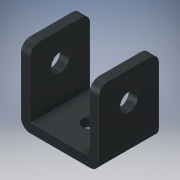
# Autodesk Inventor part: linear_actuator_connector
Saved by Autodesk Inventor 2019.4 (Build 234330000, 330)
## iProperties
Created: 2020-09-27
Part Number: linear_actuator_connector
Material: Iron, Cast
Document SubType Name: Modeling
Designer: deanv
Density: 7.15 g/cm^3
Appearance: Iron Gray
Author: deanv
Autodesk Inventor part; units mm, degrees
ref_plane "YZ Plane" through (0, 0, 0) normal (1, 0, 0) x (0, 1, 0)
ref_plane "XZ Plane" through (0, 0, 0) normal (0, 1, 0) x (-1, 0, 0)
ref_plane "XY Plane" through (0, 0, 0) normal (0, 0, 1) x (1, 0, 0)
sketch "Sketch1" plane through (0, 0, 0) normal (0, 0, 1) x (1, 0, 0)
  line L0 (-13, -12.5) -> (13, -12.5) construction
  line L1 (13, -12.5) -> (13, 12.5) construction
  line L2 (13, 12.5) -> (-13, 12.5) construction
  line L3 (-13, 12.5) -> (-13, -12.5) construction
  line L4 (-13, -12.5) -> (13, 12.5) construction
  line L5 (13, -12.5) -> (-13, 12.5) construction
  line L6 (-10, 12.5) -> (10, 12.5) construction
  line L7 (10, 12.5) -> (10, -9.5) construction
  line L8 (10, -9.5) -> (-10, -9.5) construction
  line L9 (-10, -9.5) -> (-10, 12.5) construction
  line L10 (-10, 12.5) -> (-13, 12.5)
  line L11 (-13, 12.5) -> (-13, -12.5)
  line L12 (-13, -12.5) -> (13, -12.5)
  line L13 (13, -12.5) -> (13, 12.5)
  line L14 (13, 12.5) -> (10, 12.5)
  line L15 (10, 12.5) -> (10, -9.5)
  line L16 (10, -9.5) -> (-10, -9.5)
  line L17 (-10, -9.5) -> (-10, 12.5)
  point P0 (0, 0)
  dimension "d0" = 26
  dimension "d1" = 25
  dimension "d2" = 3
  dimension "d3" = 3
  dimension "d4" = 3
  constraints: 36 end point, 5 collinear, 5 perpendicular, 4 parallel, 2 horizontal, 2 midpoint, 1 point on line
  measures "d0" distance of L2.end L1.end
  measures "d1" distance of L1.end L0.end
  measures "d2" distance between parallel lines of L3 L9
  measures "d3" distance between parallel lines of L1 L7
  measures "d4" distance between parallel lines of L0 L8
extrude "Extrusion1" add sketch "Sketch1" along normal blind 20
sketch "Sketch2" plane through (13, -12.5, 0) normal (1, 0, 0) x (0, 0, -1)
  line L0 (-20, 25) -> (-20, 0) construction
  line L1 (0, 0) -> (0, 25) construction
  line L2 (-20, 25) -> (0, 25) construction
  line L3 (0, 25) -> (0, 5) construction
  line L4 (0, 5) -> (-20, 5) construction
  line L5 (-20, 5) -> (-20, 25) construction
  line L6 (-20, 25) -> (0, 5) construction
  line L7 (-20, 5) -> (0, 25) construction
  line L8 (0, 25) -> (-20, 25) construction
  line L9 (-10, 25) -> (-10, 5) construction
  circle A0 centre (-10, 15.5) radius 3
  line L10 (0, 25) -> (0, 0) projected
  line L11 (-20, 0) -> (0, 0) construction
  line L12 (0, 0) -> (0, 3) construction
  line L13 (0, 3) -> (-20, 3) construction
  line L14 (-20, 3) -> (-20, 0) construction
  point P0 (0, 12.5)
  dimension "d7" = 20
  dimension "d17" = 6
  dimension "d20" = 3
  dimension "d21" = 12.5
  constraints: 22 end point, 4 parallel, 3 point on line, 2 horizontal, 2 midpoint, 2 perpendicular, 1 centre point
  measures "d7" distance of L2.end L3.end
  measures "d17" diameter of A0
  measures "d20" distance of L12.end L11.end
  measures "d21" distance from line of L13 A0.centre
extrude "Extrusion2" cut sketch "Sketch2" against normal blind 39
sketch "Sketch3" plane through (-13, -12.5, 0) normal (0, -1, 0) x (1, 0, 0)
  line L0 (0, 20) -> (26, 0) construction
  line L1 (0, 0) -> (26, 20) construction
  circle A0 centre (13, 10) radius 2.5
  point P0 (13, 0)
  dimension "d11" = 5
  constraints: 4 end point, 1 centre point, 1 midpoint
  measures "d11" diameter of A0
extrude "Extrusion3" cut sketch "Sketch3" against normal blind 39
fillet "Fillet2" radius 3 2 edges at (13, -12.5, 10) (-13, -12.5, 10)
fillet "Fillet3" radius 3 4 edges at (-11.5, 12.5, 20) (-11.5, 12.5, 0) (11.5, 12.5, 20) (11.5, 12.5, 0)
equation "\"d3\" = d2"
equation "\"d4\" = d3"
body "Solid1"
